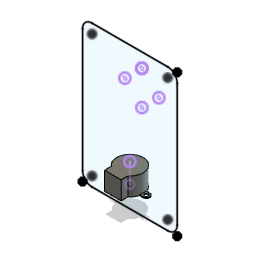
stepper mount v8 (Autodesk Fusion 360 design; units mm, degrees)
Autodesk Fusion 360 part; units mm, degrees
sketch "motor face" plane through (0, 0, 0) normal (0, 1, 0) x (1, 0, 0)
  circle A0 centre (0, 0) radius 14
  line L0 (0, 0) -> (37.538, 0) construction
  circle A1 centre (17.5, 0) radius 2
  line L1 (17.5, 3.5) -> (13.5554, 3.5)
  line L2 (17.5, -3.5) -> (13.5554, -3.5)
  line L3 (0, 0) -> (0, 22.7217) construction
  circle A2 centre (0, 8) radius 4.5
  circle A3 centre (-17.5, 0) radius 2
  line L4 (-17.5, 3.5) -> (-13.5554, 3.5)
  line L5 (-17.5, -3.5) -> (-13.5554, -3.5)
  arc A4 (17.5, -3.5) -> (17.5, 3.5) centre (17.5, 0) ccw
  arc A5 (-17.5, 3.5) -> (-17.5, -3.5) centre (-17.5, 0) ccw
  line L6 (0, 0) -> (0, -28.4127) construction
  line L7 (0, -18) -> (8.8, -18)
  line L8 (8.8, -18) -> (8.8, -10.8885)
  line L9 (-8.8, -18) -> (-8.8, -10.8885)
  line L10 (0, -18) -> (-8.8, -18)
  circle A6 centre (0, 8) radius 2.46
  line L11 (-0.98, 10.2564) -> (-0.98, 5.7436)
  line L12 (0.98, 10.2564) -> (0.98, 5.7436)
  point P0 (0, 14)
  point P1 (0, 3.5)
  dimension "d1" = 28
  dimension "d2" = 4
  dimension "d3" = 17.5
  dimension "d4" = 7
  dimension "d5" = 9
  dimension "d6" = 10.5
  dimension "d7" = 8.8
  dimension "d8" = 32
  dimension "d11" = 4.92
  dimension "d12" = 0.98
  constraint coincident A0.centre L0.start
  constraint horizontal L0
  constraint coincident L0 A1.centre
  constraint concentric A1 A4
  constraint coincident A0 L1.end
  constraint tangent L1 A4
  constraint horizontal L1
  constraint coincident A0 L2.end
  constraint tangent L2 A4
  constraint parallel L1 L2
  constraint perpendicular L0 L3
  constraint coincident L3 A2.centre
  constraint coincident A0 P0
  constraint coincident L3 P0
  constraint coincident A2 P1
  constraint coincident L3 P1
  constraint symmetric A1 L3 A3
  constraint symmetric L3 A4 A5
  constraint symmetric L1.start L3 L4.start
  constraint symmetric L1.end L3 L4.end
  constraint symmetric L2.start L3 L5.start
  constraint symmetric L2.end L3 L5.end
  constraint perpendicular L0 L6
  constraint coincident L6 L7.start
  constraint perpendicular L6 L7
  constraint coincident A0 L8.end
  constraint perpendicular L7 L8
  constraint symmetric L6 L7.start L10.start
  constraint symmetric L6 L7.end L9.start
  constraint symmetric L6 L8.end L9.end
  constraint concentric A2 A6
  constraint coincident A6 L11.start
  constraint coincident A6 L11.end
  constraint vertical L11
  constraint symmetric L3 L11.start L12.start
  constraint symmetric L3 L11.end L12.end
  measures "d1" diameter of A0
  measures "d2" diameter of A1
  measures "d3" distance of A0.centre A1.centre
  measures "d4" diameter of A4
  measures "d5" diameter of A2
  measures "d6" distance of P0 P1
  measures "d7" distance of L7.start L7.end
  measures "d8" distance of P0 L7
  measures "d11" diameter of A6
  measures "d12" distance of L3 L11
extrude "Extrude1" add sketch "motor face" along normal blind 19.3 contours A0 | A0 L7 L8 L9 L10 | A2 | A6 L12 | A6 L11 L12 | A6 L11 makes body 1
extrude "Extrude2" add sketch "motor face" along normal blind 0.8 contours A0 L1 L2 A4 | A0 L4 L5 A5 bodies 1
extrude "Extrude3" add sketch "motor face" against normal blind 1.34 contours A2 | A6 L12 | A6 L11 L12 | A6 L11 bodies 1
extrude "Extrude4" add sketch "motor face" against normal blind 3.43 contours A6 L12 | A6 L11 L12 | A6 L11 bodies 1
extrude "Extrude5" add sketch "motor face" against normal blind 9.43 contours A6 L11 L12 bodies 1
sketch "motor clamp face" plane through (0, 0, 0) normal (0, 1, 0) x (1, 0, 0)
  circle A0 centre (17.5, 0) radius 2
  line L0 (17.5, 3.5) -> (13.5554, 3.5)
  arc A1 (17.5, -3.5) -> (17.5, 3.5) centre (17.5, 0) ccw
  line L1 (17.5, -3.5) -> (13.5554, -3.5)
  arc A2 (13.5554, 3.5) -> (-13.5554, 3.5) centre (0, 0) ccw
  arc A3 (-13.5554, -3.5) -> (-8.8, -10.8885) centre (0, 0) ccw
  arc A4 (8.8, -10.8885) -> (13.5554, -3.5) centre (0, 0) ccw
  circle A5 centre (-17.5, 0) radius 2
  line L2 (-17.5, -3.5) -> (-13.5554, -3.5)
  arc A6 (-17.5, 3.5) -> (-17.5, -3.5) centre (-17.5, 0) ccw
  line L3 (-17.5, 3.5) -> (-13.5554, 3.5)
  line L4 (8.8, -18) -> (-8.8, -18)
  line L5 (-8.8, -18) -> (-8.8, -10.8885)
  line L6 (8.8, -18) -> (8.8, -10.8885)
  circle A7 centre (0, 0) radius 22
  line L7 (-22, 10) -> (22, 10)
  line L8 (22, 10) -> (22, -10)
  line L9 (22, -10) -> (-22, -10)
  line L10 (-22, -10) -> (-22, 10)
  line L11 (-22, 10) -> (22, -10) construction
  line L12 (22, 10) -> (-22, -10) construction
  circle A8 centre (17.5, 0) radius 1.25
  circle A9 centre (-17.5, 0) radius 1.25
  dimension "d21" = 20
  dimension "d25" = 44
  dimension "d27" = 2.5
  dimension "d28" = 2.5
  constraint concentric A2 A7
  constraint horizontal L7
  constraint perpendicular L7 L8
  constraint parallel L7 L9
  constraint parallel L8 L10
  constraint coincident L11 A2.centre
  constraint coincident L12 A2.centre
  constraint coincident A2.centre A3.centre
  constraint tangent A7 L10
  constraint concentric A0 A8
  constraint concentric A5 A9
  measures "d21" distance of L7.end L8.end
  measures "d25" distance of L7.start L7.end
  measures "d27" diameter of A8
  measures "d28" diameter of A9
extrude "Extrude6" add sketch "motor clamp face" along normal blind 40 separate body contours A0 | L0 A1 L1 A2 A3 A4 L2 A6 L3 L7 L9 | L0 A1 L1 A2 A4 A7 L7 L9 | A2 A3 L2 A6 L3 A7 L7 L9 | A5 | A8 | A9 makes body 2
combine "Combine1" operation cut target body 2 tool bodies 1 keep tools
move_face "OffsetFaces1" offset -0.3 9 faces at (12.7902, 12.8667, 5.6931) (-3.266, 19.3, -3.3333) (16.1851, 0.2667, 3.5) (19.325, 0.2667, -2.9865) (16.1851, 0.2667, -3.5) (-12.7902, 12.8667, -5.6931) (-16.1851, 0.2667, -3.5) (-19.325, 0.2667, 2.9865) (-16.1851, 0.2667, 3.5) on bodies 2
move_face "OffsetFaces2" offset -0.8 2 faces at (-16.9788, 0, -0.179) (18.1667, 0, 0.5785) on bodies 2
extrude "Extrude7" cut sketch "motor clamp face" along normal blind 20 contours A8 | A9 bodies 2
sketch "bar clamp face" plane through (0, 40, 0) normal (0, 1, 0) x (-1, 0, 0)
  arc A0 (19.5959, -10) -> (19.5959, 10) centre (0, 0) ccw
  line L0 (19.5959, 10) -> (-19.5959, 10)
  arc A1 (-19.5959, 10) -> (-19.5959, -10) centre (0, 0) ccw
  line L1 (-19.5959, -10) -> (19.5959, -10)
  line L2 (-6.35, 6.35) -> (6.35, 6.35)
  line L3 (6.35, 6.35) -> (6.35, -6.35)
  line L4 (6.35, -6.35) -> (-6.35, -6.35)
  line L5 (-6.35, -6.35) -> (-6.35, 6.35)
  line L6 (-6.35, 6.35) -> (6.35, -6.35) construction
  line L7 (6.35, 6.35) -> (-6.35, -6.35) construction
  line L8 (-22, 0.5) -> (22, 0.5)
  line L9 (22, 0.5) -> (22, -0.5)
  line L10 (22, -0.5) -> (-22, -0.5)
  line L11 (-22, -0.5) -> (-22, 0.5)
  line L12 (-22, 0.5) -> (22, -0.5) construction
  line L13 (22, 0.5) -> (-22, -0.5) construction
  dimension "d33" = 12.7
  dimension "d34" = 12.7
  dimension "d35" = 1
  constraint horizontal L2
  constraint perpendicular L2 L3
  constraint parallel L2 L4
  constraint parallel L3 L5
  constraint coincident L6 A0.centre
  constraint coincident L7 A0.centre
  constraint coincident A0.centre A1.centre
  constraint horizontal L8
  constraint perpendicular L8 L9
  constraint parallel L8 L10
  constraint parallel L9 L11
  constraint coincident L12 A0.centre
  constraint coincident L13 A0.centre
  constraint tangent A1 L11
  measures "d33" distance of L3.end L4.end
  measures "d34" distance of L2.end L3.end
  measures "d35" distance of L8.end L9.end
extrude "Extrude8" cut sketch "bar clamp face" against normal up to surface (20.4 mm away) contours A0 L3 L8 L10 | L3 L5 L8 L10 | L3 L4 L5 L10 | A1 L5 L8 L10 | L2 L3 L5 L8 bodies 2
sketch "bar clamp bolts" plane through (0, 0, -10) normal (0, 0, -1) x (-1, 0, 0)
  line L0 (-10.222, 0) -> (-10.222, 19.6)
  line L1 (-10.222, 19.6) -> (10.222, 19.6)
  line L2 (10.222, 19.6) -> (10.222, 0)
  line L3 (10.222, 0) -> (19.5959, 0)
  line L4 (19.5959, 0) -> (19.5959, 40)
  line L5 (19.5959, 40) -> (-19.5959, 40)
  line L6 (-19.5959, 40) -> (-19.5959, 0)
  line L7 (-19.5959, 0) -> (-10.222, 0)
  line L8 (-6.35, 19.6) -> (6.35, 19.6)
  line L9 (6.35, 19.6) -> (6.35, 40)
  line L10 (6.35, 40) -> (-6.35, 40)
  line L11 (-6.35, 40) -> (-6.35, 19.6)
  circle A0 centre (-11.4931, 31) radius 1.6
  circle A1 centre (-11.4931, 31) radius 3
  line L12 (-11.4931, 31) -> (-11.4931, 34) construction
  line L13 (-11.4931, 31) -> (-8.35, 31) construction
  line L14 (0, 1.75) -> (0, 22.5)
  circle A2 centre (11.4931, 31) radius 1.6
  circle A3 centre (11.4931, 31) radius 3
  point P0 (-8.4931, 31)
  point P1 (-11.4931, 34)
  dimension "d38" = 3.2
  dimension "d39" = 6
  dimension "d40" = 6
  dimension "d41" = 2
  constraint concentric A0 A1
  constraint coincident A0.centre A1.centre
  constraint coincident A1 P1
  constraint vertical L12
  constraint perpendicular L12 L13
  constraint coincident A1 P0
  constraint coincident L13 P0
  constraint coincident P1 L12.end
  constraint symmetric A0 L14 A2
  constraint symmetric A1 L14 A3
  measures "d38" diameter of A0
  measures "d39" diameter of A1
  measures "d40" distance of L5 P1
  measures "d41" distance of L11 L13.end
extrude "Extrude9" cut sketch "bar clamp bolts" against normal up to surface (20 mm away) contours A0 | A2 bodies 2
extrude "Extrude10" cut sketch "bar clamp bolts" against normal blind 1 contours A1 | A3 bodies 2
sketch "bar clamp nuts" plane through (0, 0, 10) normal (0, 0, 1) x (1, 0, 0)
  circle A0 centre (11.4931, 31) radius 1.6
  circle A1 centre (-11.4931, 31) radius 1.6
  line L0 (10.222, 19.6) -> (10.222, 0)
  line L1 (10.222, 0) -> (19.5959, 0)
  line L2 (19.5959, 0) -> (19.5959, 40)
  line L3 (19.5959, 40) -> (-19.5959, 40)
  line L4 (-19.5959, 40) -> (-19.5959, 0)
  line L5 (-19.5959, 0) -> (-10.222, 0)
  line L6 (-10.222, 0) -> (-10.222, 19.6)
  line L7 (-10.222, 19.6) -> (10.222, 19.6)
  circle A2 centre (-11.4931, 31) radius 3
  circle A3 centre (11.4931, 31) radius 3
  dimension "d46" = 6
  dimension "d47" = 6
  constraint concentric A1 A2
  constraint concentric A0 A3
  measures "d46" diameter of A2
  measures "d47" diameter of A3
extrude "Extrude11" cut sketch "bar clamp nuts" against normal blind 1 contours A2 | A3 bodies 2
chamfer "Chamfer1" distance 1 angle 45 6 edges at (0, 40, -6.35) (-6.35, 40, -3.425) (6.35, 40, -3.425) (6.35, 40, 3.425) (0, 40, 6.35) (-6.35, 40, 3.425) on bodies 2
fillet "Fillet1" radius 4 10 edges at (19.5959, 20, -10) (-19.5959, 20, -10) (0, 40, -10) (19.5959, 20, 10) (21.3307, 40, 5.3852) (21.3307, 40, -5.3852) (0, 40, 10) (-19.5959, 20, 10) (-21.3307, 40, -5.3852) (-21.3307, 40, 5.3852) on bodies 2
extrude "Extrude12" add sketch "bar clamp face" along normal blind 100 separate body contours L3 L5 L8 L10 | L3 L4 L5 L10 | L2 L3 L5 L8 makes body 3
sketch "v bar" plane through (0, 0, 6.35) normal (0, 0, 1) x (1, 0, 0)
  line L0 (-6.35, 40) -> (6.35, 40)
  line L1 (6.35, 40) -> (6.35, 140)
  line L2 (6.35, 140) -> (-6.35, 140)
  line L3 (-6.35, 140) -> (-6.35, 40)
  line L4 (19.05, 90) -> (6.35, 90)
  line L5 (6.35, 90) -> (6.35, 102.7)
  line L6 (6.35, 102.7) -> (19.05, 102.7)
  line L7 (19.05, 102.7) -> (19.05, 90)
  line L8 (19.05, 90) -> (6.35, 102.7) construction
  line L9 (6.35, 90) -> (19.05, 102.7) construction
  line L10 (6.35, 40) -> (-6.35, 40)
  point P0 (12.7, 96.35)
  dimension "d55" = 12.7
  dimension "d56" = 12.7
  dimension "d57" = 50
  constraint horizontal L4
  constraint perpendicular L4 L5
  constraint parallel L4 L6
  constraint parallel L5 L7
  constraint coincident L8 P0
  constraint coincident L9 P0
  constraint collinear L1 L5
  measures "d55" distance of L5.end L6.end
  measures "d56" distance of L4.end L5.end
  measures "d57" distance of L4 L10
extrude "Extrude13" add sketch "v bar" along normal mid plane 100 separate body contours L1 L4 L5 L6 L7 makes body 4
sketch "A clamp bolts" plane through (6.35, 0, 0) normal (1, 0, 0) x (0, 0, -1)
  line L0 (-6.35, 40) -> (6.35, 40)
  line L1 (6.35, 40) -> (6.35, 140)
  line L2 (6.35, 140) -> (-6.35, 140)
  line L3 (-6.35, 140) -> (-6.35, 40)
  line L4 (43.65, 102.7) -> (-56.35, 102.7)
  line L5 (-56.35, 102.7) -> (-56.35, 90)
  line L6 (-56.35, 90) -> (43.65, 90)
  line L7 (43.65, 90) -> (43.65, 102.7)
  circle A0 centre (11.35, 107.7) radius 3 construction
  circle A1 centre (11.35, 107.7) radius 1.6
  line L8 (6.35, 112.7) -> (16.35, 112.7)
  line L9 (16.35, 112.7) -> (16.35, 102.7)
  line L10 (0, 40) -> (0, 140) construction
  line L11 (-56.35, 96.35) -> (43.65, 96.35) construction
  line L12 (-6.35, 112.7) -> (-16.35, 112.7)
  line L13 (-16.35, 112.7) -> (-16.35, 102.7)
  circle A2 centre (-11.35, 107.7) radius 1.6
  circle A3 centre (-11.35, 85) radius 1.6
  line L14 (-6.35, 80) -> (-16.35, 80)
  line L15 (-16.35, 80) -> (-16.35, 90)
  line L16 (6.35, 80) -> (16.35, 80)
  circle A4 centre (11.35, 85) radius 1.6
  line L17 (16.35, 80) -> (16.35, 90)
  line L18 (6.35, 112.7) -> (-6.35, 112.7)
  line L19 (16.35, 102.7) -> (16.35, 90)
  line L20 (6.35, 80) -> (-6.35, 80)
  line L21 (-16.35, 102.7) -> (-16.35, 90)
  circle A5 centre (-11.35, 107.7) radius 3
  circle A6 centre (11.35, 85) radius 3
  line L22 (-14.1, 83.4123) -> (-11.35, 81.8246)
  line L23 (-11.35, 81.8246) -> (-8.6, 83.4123)
  line L24 (-8.6, 83.4123) -> (-8.6, 86.5877)
  line L25 (-8.6, 86.5877) -> (-11.35, 88.1754)
  line L26 (-11.35, 88.1754) -> (-14.1, 86.5877)
  line L27 (-14.1, 86.5877) -> (-14.1, 83.4123)
  line L28 (8.6, 106.1123) -> (11.35, 104.5246)
  line L29 (11.35, 104.5246) -> (14.1, 106.1123)
  line L30 (14.1, 106.1123) -> (14.1, 109.2877)
  line L31 (14.1, 109.2877) -> (11.35, 110.8754)
  line L32 (11.35, 110.8754) -> (8.6, 109.2877)
  line L33 (8.6, 109.2877) -> (8.6, 106.1123)
  point P0 (8.35, 107.7)
  point P1 (11.35, 104.7)
  point P2 (11.35, 110.7)
  point P3 (14.35, 107.7)
  point P4 (-11.35, 85)
  point P5 (11.35, 107.7)
  dimension "d60" = 6
  dimension "d61" = 3.2
  dimension "d62" = 2
  dimension "d63" = 2
  dimension "d64" = 2
  dimension "d65" = 2
  dimension "d71" = 6
  dimension "d72" = 6
  dimension "d73" = 2.75
  dimension "d74" = 2.75
  constraint concentric A0 A1
  constraint coincident A0 P0
  constraint coincident A0 P1
  constraint coincident L1 L8.start
  constraint perpendicular L1 L8
  constraint coincident L4 L9.end
  constraint perpendicular L4 L9
  constraint coincident A0 P2
  constraint coincident A0 P3
  constraint midpoint L0 L10.start
  constraint midpoint L2 L10.end
  constraint midpoint L5 L11.start
  constraint midpoint L7 L11.end
  constraint symmetric A1 L10 A2
  constraint symmetric L8.start L10 L12.start
  constraint symmetric L8.end L10 L12.end
  constraint symmetric L9.end L10 L13.end
  constraint symmetric A1 L11 A4
  constraint symmetric L8.start L11 L16.start
  constraint symmetric L8.end L11 L16.end
  constraint symmetric L9.end L11 L17.end
  constraint symmetric L11 L12.start L14.start
  constraint symmetric L11 L12.end L14.end
  constraint symmetric L11 L13.end L15.end
  constraint symmetric L11 A2 A3
  constraint concentric A2 A5
  constraint concentric A4 A6
  constraint coincident P4 A3.centre
  constraint coincident P5 A0.centre
  measures "d60" diameter of A0
  measures "d61" diameter of A1
  measures "d62" distance of L1 P0
  measures "d63" distance of L4 P1
  measures "d64" distance of L9 P3
  measures "d65" distance of L8 P2
  measures "d71" diameter of A5
  measures "d72" diameter of A6
  measures "d73" distance of P4 L27
  measures "d74" distance of P5 L33
extrude "Extrude14" add sketch "A clamp bolts" along normal blind 15.7 separate body contours L3 L6 L14 L15 | L1 L3 L6 L20 | L1 L6 L16 L17 | L3 L4 L6 L21 | L1 L3 L4 L6 | L1 L4 L6 L19 | L3 L4 L12 L13 | L1 L3 L4 L18 | L1 L4 L8 L9 | A5 | A6 | L22 L23 L24 L25 L26 L27 | L28 L29 L30 L31 L32 L33 makes body 5
combine "Combine2" operation cut target body 5 tool bodies 4 keep tools
move_face "OffsetFaces3" offset -0.3 2 faces at (6.35, 81.1702, 3.5885) (6.35, 103.8702, 3.5885) on bodies 5
fillet "Fillet2" radius 3 8 edges at (14.35, 112.7, 16.35) (22.05, 96.35, 16.35) (22.05, 112.7, 0) (22.05, 80, 0) (14.35, 80, 16.35) (14.35, 80, -16.35) (22.05, 96.35, -16.35) (14.35, 112.7, -16.35) on bodies 5
extrude "Extrude15" cut sketch "A clamp bolts" along normal blind 20 from surface at 11 contours A5 | A6 | L22 L23 L24 L25 L26 L27 | L28 L29 L30 L31 L32 L33 bodies 5
mirror "Mirror1" about plane through (6.35, 90, 6.35) normal (-1, 0, 0) of bodies 5 makes body 6
sketch "B clamp" plane through (6.35, 0, 0) normal (-1, 0, 0) x (0, 0, 1)
  line L0 (-43.65, 90) -> (56.35, 90)
  line L1 (56.35, 90) -> (56.35, 102.7)
  line L2 (56.35, 102.7) -> (-43.65, 102.7)
  line L3 (-43.65, 102.7) -> (-43.65, 90)
  line L4 (-43.65, 102.7) -> (-43.65, 90)
  line L5 (56.35, 102.7) -> (-43.65, 102.7)
  line L6 (56.35, 90) -> (56.35, 102.7)
  line L7 (-43.65, 90) -> (56.35, 90)
  line L8 (-6.35, 40) -> (6.35, 40)
  line L9 (-6.35, 40) -> (-6.35, 140)
  line L10 (6.35, 140) -> (-6.35, 140)
  line L11 (6.35, 40) -> (6.35, 140)
  circle A0 centre (9.35, 105.7) radius 3
  line L12 (-43.65, 96.35) -> (56.35, 96.35) construction
  line L13 (0, 140) -> (0, 40) construction
  line L14 (0, 96.35) -> (49.0077, 47.3423) construction
  line L15 (9.8855, 86.4645) -> (35.4058, 111.9847)
  line L16 (0, 96.35) -> (34.5073, 130.8573) construction
  line L17 (15.0069, 111.3569) -> (24.8924, 101.4713)
  circle A1 centre (9.35, 105.7) radius 1.6
  circle A2 centre (9.35, 105.7) radius 1.1
  line L18 (-9.8855, 106.2355) -> (15.6347, 131.7558)
  line L19 (15.0069, 111.3569) -> (5.1213, 121.2424)
  line L20 (9.8855, 86.4645) -> (-15.6347, 60.9442)
  line L21 (-15.0069, 81.3431) -> (-5.1213, 71.4576)
  line L22 (-9.8855, 106.2355) -> (-35.4058, 80.7153)
  circle A3 centre (-9.35, 87) radius 3
  circle A4 centre (-9.35, 87) radius 1.6
  circle A5 centre (-9.35, 87) radius 1.1
  line L23 (-15.0069, 81.3431) -> (-24.8924, 91.2287)
  point P0 (6.35, 90)
  point P1 (9.8855, 86.4645)
  dimension "d80" = 6
  dimension "d81" = 135
  dimension "d82" = 5
  dimension "d83" = 8
  dimension "d84" = 3.2
  dimension "d85" = 2.2
  constraint tangent L11 A0
  constraint tangent L2 A0
  constraint midpoint L4 L12.start
  constraint midpoint L6 L12.end
  constraint midpoint L10 L13.start
  constraint midpoint L8 L13.end
  constraint coincident L12 L14.start
  constraint coincident L13 L14.start
  constraint coincident L14 P1
  constraint perpendicular L14 L15
  constraint midpoint L7 P0
  constraint coincident P1 L15.start
  constraint perpendicular L14 L16
  constraint coincident L16 L17.start
  constraint coincident L15 L17.end
  constraint perpendicular L15 L17
  constraint concentric A0 A1
  constraint concentric A1 A2
  constraint symmetric P1 L16 L18.start
  constraint symmetric L15.end L16 L18.end
  constraint symmetric L16 L17.start L19.start
  constraint symmetric L16 L17.end L19.end
  constraint symmetric A0 L14 A3
  constraint symmetric L14 P1 L15.start
  constraint symmetric L14 L15.end L20.end
  constraint symmetric L14 L17.start L21.start
  constraint symmetric L14 L17.end L21.end
  constraint symmetric L14 A1 A4
  constraint symmetric L14 A2 A5
  constraint symmetric L14 L18.start L22.start
  constraint symmetric L14 L18.end L22.end
  constraint symmetric L14 L19.end L23.end
  measures "d80" diameter of A0
  measures "d81" angle of L13 L14
  measures "d82" distance of P0 P1
  measures "d83" distance of A0.centre L17.start
  measures "d84" diameter of A1
  measures "d85" diameter of A2
extrude "Extrude16" add sketch "B clamp" along normal blind 15.7 separate body contours L0 L2 L5 L7 L9 L22 L23 | L0 L7 L9 L21 A3 L23 | L2 L5 L9 L18 L22 | L0 L7 L9 A3 | A3 | L2 L5 L9 L11 L18 L19 | L0 L2 L5 L7 L9 L11 | L0 L7 L9 L11 L20 L21 | L2 L5 L11 A0 | L0 L2 L5 L7 L11 L15 L17 | L0 L7 L11 L15 L20 | L2 L5 L11 A0 L17 L19 | A0 | A1 makes body 7
combine "Combine3" operation cut target body 7 tool bodies 3 keep tools
extrude "Extrude19" add sketch "B clamp" against normal blind 3.175 contours L0 L7 L9 L21 A3 L23 | L0 L7 L9 A3 | A3 | A4 | A5 bodies 7
extrude "Extrude20" cut sketch "B clamp" along normal blind 4.175 contours L2 L5 L11 A0 | L2 L5 L11 A0 L17 L19 | A0 | A1 | A2 bodies 7
extrude "Extrude21" cut sketch "B clamp" against normal blind 10 from surface at 15.7 contours A3 | A4 | A5 bodies 7
extrude "Extrude22" cut sketch "B clamp" along normal mid plane 100 contours A4 | A5 bodies 7
fillet "Fillet3" radius 3 6 edges at (-9.35, 106.2355, -9.8855) (-9.35, 86.4645, 9.8855) (-9.35, 111.3569, 15.0069) (-9.35, 81.3431, -15.0069) (-1.5, 101.4713, 24.8924) (-1.5, 91.2287, -24.8924) on bodies 7
sketch "base clamp layout" plane through (0, 0, 56.35) normal (0, 0, 1) x (1, 0, 0)
  line L0 (19.05, 102.7) -> (6.35, 102.7)
  line L1 (6.35, 102.7) -> (6.35, 90)
  line L2 (6.35, 90) -> (19.05, 90)
  line L3 (19.05, 90) -> (19.05, 102.7)
  line L4 (6.35, 102.7) -> (19.05, 102.7)
  line L5 (19.05, 102.7) -> (19.05, 90)
  line L6 (19.05, 90) -> (6.35, 90)
  line L7 (6.35, 90) -> (6.35, 102.7)
  line L8 (19.05, 102.7) -> (-29.3857, 54.2643) construction
  line L9 (19.05, 102.7) -> (87.5484, 102.7) construction
  line L10 (19.05, 90) -> (6.35, 102.7) construction
  circle A0 centre (12.7, 96.35) radius 14.9803
  line L11 (4.9358, 88.5858) -> (-2.2698, 95.7914) construction
  line L12 (1.5459, 86.3503) -> (22.6997, 107.5041)
  line L13 (12.7, 96.35) -> (-15.2309, 96.35) construction
  circle A1 centre (-5.2803, 96.35) radius 3 construction
  circle A2 centre (-5.2803, 96.35) radius 1.6
  circle A3 centre (12.7, 114.3303) radius 1.6
  circle A4 centre (12.7, 96.35) radius 20.9803
  line L14 (1.5459, 86.3503) -> (-5.9226, 78.8819)
  line L15 (22.6997, 107.5041) -> (30.5569, 115.3614)
  circle A5 centre (12.7, 78.3697) radius 1.6
  circle A6 centre (30.6803, 96.35) radius 1.6
  point P0 (2.1074, 85.7574)
  point P1 (4.9358, 88.5858)
  dimension "d105" = 135
  dimension "d106" = 2
  dimension "d107" = 4
  dimension "d120" = 6
  dimension "d121" = 3.2
  constraint horizontal L9
  constraint coincident L0.start L3.end
  constraint coincident L2.end L3.start
  constraint coincident L0.end L1.start
  constraint midpoint L10 A0.centre
  constraint coincident L8 P1
  constraint coincident A0 L11.end
  constraint perpendicular L8 L11
  constraint coincident A0 P0
  constraint coincident L8 P0
  constraint coincident P1 L11.start
  constraint coincident A0 L12.start
  constraint coincident A0 L12.end
  constraint perpendicular L10 L12
  constraint coincident A0.centre L13.start
  constraint horizontal L13
  constraint coincident L13 A1.centre
  constraint tangent A0 A1
  constraint concentric A1 A2
  constraint symmetric L10 A2 A3
  constraint concentric A0 A4
  constraint tangent A1 A4
  constraint parallel L12 L14
  constraint parallel L12 L15
  constraint symmetric L8 A2 A5
  constraint symmetric L8 A3 A6
  measures "d105" angle of L8 L9
  measures "d106" distance of L1.end P1
  measures "d107" distance of P0 P1
  measures "d120" diameter of A1
  measures "d121" diameter of A2
extrude "Extrude23" add sketch "base clamp layout" against normal blind 12 separate body contours L0 L1 L4 L7 A0 L12 makes body 8
sketch "base clamp bolts" plane through (-42.4022, 42.4022, 0) normal (0.707107, -0.707107, 0) x (0, 0, -1)
  line L0 (-56.35, 68.9461) -> (-56.35, 62.152)
  line L1 (-56.35, 62.152) -> (-44.35, 62.152)
  line L2 (-44.35, 62.152) -> (-44.35, 68.9461)
  line L3 (-44.35, 68.9461) -> (-56.35, 68.9461)
  line L4 (-56.35, 66.1297) -> (-44.35, 66.1297) construction
  circle A0 centre (-50.35, 66.1297) radius 1.6
  circle A1 centre (-50.35, 66.1297) radius 3
  circle A2 centre (-50.35, 66.1297) radius 1.1
  line L5 (-56.35, 77.11) -> (-43.0331, 77.11) construction
  circle A3 centre (-50.35, 88.0903) radius 1.1
  point P0 (-56.35, 66.1297)
  point P1 (-56.35, 66.1297)
  point P2 (-50.35, 66.1297)
  point P3 (-56.35, 77.11)
  dimension "d110" = 3.2
  dimension "d111" = 6
  dimension "d112" = 2.2
  constraint coincident P1 P0
  constraint coincident L2 L4.end
  constraint perpendicular L2 L4
  constraint midpoint L4 P2
  constraint coincident P2 A0.centre
  constraint concentric A0 A1
  constraint concentric A1 A2
  constraint coincident P3 L5.start
  constraint horizontal L5
  constraint symmetric A2 L5 A3
  measures "d110" diameter of A0
  measures "d111" diameter of A1
  measures "d112" diameter of A2
extrude "Extrude24" cut sketch "base clamp bolts" against normal blind 30 contours A3 bodies 8
extrude "Extrude25" cut sketch "base clamp bolts" against normal blind 30 contours A0 | A2 bodies 8
extrude "Extrude27" add sketch "base clamp layout" against normal blind 3 contours A0 A4 L14 L15 picked at (-4.69, 92.2283) bodies 8
fillet "Fillet4" radius 3 1 edges at (2.1074, 106.9426, 53.35) on bodies 8
extrude "Extrude26" cut sketch "base clamp bolts" against normal blind 20 from surface at -5 contours L3 A1 | L3 A1 bodies 8
sketch "Base bolt counterbores" plane through (0, 0, 53.35) normal (0, 0, -1) x (-1, 0, 0)
  arc A0 (2.7013, 82.1032) -> (-26.9468, 111.7513) centre (-12.7, 96.35) ccw
  line L0 (-26.9468, 111.7513) -> (-24.8236, 109.6281)
  arc A1 (-14.2984, 114.2591) -> (-24.8236, 109.6281) centre (-12.7, 96.35) ccw
  arc A2 (-11.1016, 114.2591) -> (-14.2984, 114.2591) centre (-12.7, 114.3303) ccw
  arc A3 (5.1321, 98.6536) -> (-11.1016, 114.2591) centre (-12.7, 96.35) ccw
  arc A4 (5.2091, 97.9484) -> (5.1321, 98.6536) centre (-12.7, 96.35) ccw
  arc A5 (5.2091, 94.7516) -> (5.2091, 97.9484) centre (5.2803, 96.35) ccw
  arc A6 (0.5781, 84.2264) -> (5.2091, 94.7516) centre (-12.7, 96.35) ccw
  line L1 (0.5781, 84.2264) -> (2.7013, 82.1032)
  circle A7 centre (-12.7, 114.3303) radius 3
  circle A8 centre (5.2803, 96.35) radius 3
  dimension "d126" = 6
  dimension "d127" = 6
  constraint concentric A2 A7
  constraint concentric A5 A8
  measures "d126" diameter of A7
  measures "d127" diameter of A8
extrude "Extrude28" cut sketch "Base bolt counterbores" along normal blind 4 contours A3 A4 A5 A6 A8 | A1 A2 A3 A7 | A3 A4 A5 A6 A8 | A1 A2 A3 A7 bodies 8
fillet "Fillet5" radius 1 2 edges at (-2.1353, 111.1853, 53.35) (2.1074, 106.9426, 44.35) on bodies 8
sketch "baseplate" plane through (0, 0, 0) normal (0, 0, 1) x (1, 0, 0)
  circle A0 centre (12.7, 78.3697) radius 1.6
  circle A1 centre (30.6803, 96.35) radius 1.6
  circle A2 centre (12.7, 114.3303) radius 1.6
  circle A3 centre (-5.2803, 96.35) radius 1.6
  line L0 (-40, -20.6697) -> (40, -20.6697)
  line L1 (50, -10.6697) -> (50, 119.3303)
  line L2 (40, 129.3303) -> (-40, 129.3303)
  line L3 (-50, 119.3303) -> (-50, -10.6697)
  line L4 (0, 1.75) -> (0, 22.5)
  arc A4 (-50, -10.6697) -> (-40, -20.6697) centre (-40, -10.6697) ccw
  arc A5 (40, -20.6697) -> (50, -10.6697) centre (40, -10.6697) ccw
  arc A6 (50, 119.3303) -> (40, 129.3303) centre (40, 119.3303) ccw
  arc A7 (-40, 129.3303) -> (-50, 119.3303) centre (-40, 119.3303) ccw
  point P0 (12.7, 114.3303)
  point P1 (-50, -20.6697)
  point P2 (50, -20.6697)
  point P3 (50, 129.3303)
  dimension "d132" = 100
  dimension "d133" = 150
  dimension "d134" = 50
  dimension "d135" = 15
  dimension "d136" = 10
  constraint horizontal L0
  constraint vertical L1
  constraint horizontal L2
  constraint vertical L3
  constraint coincident P1 L0
  constraint coincident P1 L3
  constraint tangent L0 A4
  constraint tangent L3 A4
  constraint coincident P2 L0
  constraint coincident P2 L1
  constraint tangent L0 A5
  constraint tangent L1 A5
  constraint equal A4 A5
  constraint coincident P3 L1
  constraint coincident P3 L2
  constraint tangent L1 A6
  constraint tangent L2 A6
  constraint equal A4 A6
  constraint tangent L2 A7
  constraint tangent L3 A7
  constraint equal A4 A7
  measures "d132" distance of P1 P2
  measures "d133" distance of P2 P3
  measures "d134" distance of L1 L4
  measures "d135" distance of P0 L2
  measures "d136" radius of A4
hidden bodies 2 3 4 5 6 7 8
equation "d3 = ( ( 39 - 4 ) / 2 ) * 1 mm"
equation "d7 = ( 17.6 / 2 ) * 1 mm"
equation "d12 = ( ( 4.92 - 2.96 ) / 2 ) * 1 mm"
equation "motorClearance = 0.3 mm"
equation "d26 = -motorClearance"
equation "tubeWidth = 12.7 mm"
equation "d33 = tubeWidth"
equation "d34 = tubeWidth"
equation "d55 = tubeWidth"
equation "d56 = tubeWidth"
equation "d66 = tubeWidth + 3 mm"
equation "d73 = ( 5.5 / 2 ) * 1 mm"
equation "d74 = ( 5.5 / 2 ) * 1 mm"
equation "d86 = tubeWidth + 3 mm"
equation "d94 = -tubeWidth / 4"
equation "d96 = tubeWidth / 4 + 1 mm"
named bodies: "28BYJ-48", "stepper mount", "h bar", "v bar", "A clamp1", "A clamp2", "B clamp", "base clamp"
